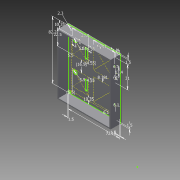
# Autodesk Inventor part: CameraCover
Saved by Autodesk Inventor 2015 (Build 190159000, 159)
## iProperties
Created: 2015-04-23
Part Number: CameraCover
Material: NylonD2W
Document SubType Name: Modeling
Designer: Akovo_000
Density: 1.13 g/cm^3
Appearance: Nylon 6
Mass: 17.9393 g
Surface Area: 219.403 cm^2
Volume: 15.8755 cm^3
Author: Akovo_000
Autodesk Inventor part; units mm, degrees
ref_plane "YZ Plane" through (0, 0, 0) normal (1, 0, 0) x (0, 1, 0)
ref_plane "XZ Plane" through (0, 0, 0) normal (0, 1, 0) x (-1, 0, 0)
ref_plane "XY Plane" through (0, 0, 0) normal (0, 0, 1) x (1, 0, 0)
sketch "Sketch1" plane through (0, 0, 0) normal (0, 1, 0) x (-1, 0, 0)
  line L0 (-58.4836, 42.7915) -> (-27.4836, 42.7915) construction
  line L1 (-27.4836, 42.7915) -> (-27.4836, 11.7915) construction
  line L2 (-27.4836, 11.7915) -> (-58.4836, 11.7915) construction
  line L3 (-58.4836, 11.7915) -> (-58.4836, 20.5915) construction
  line L4 (-58.4836, 42.7915) -> (-27.4836, 11.7915) construction
  line L5 (-27.4836, 42.7915) -> (-58.4836, 11.7915) construction
  line L6 (-58.4836, 3.6103) -> (-27.4836, 3.6103) construction
  line L7 (-27.4836, 3.6103) -> (-27.4836, -27.2085) construction
  line L8 (-27.4836, -27.2085) -> (-58.4836, -27.2085) construction
  line L9 (-58.4836, -27.2085) -> (-58.4836, -18.4991) construction
  line L10 (-58.4836, 3.6103) -> (-27.4836, -27.2085) construction
  line L11 (-20.4336, 38.5415) -> (2.0664, 38.5415) construction
  line L12 (2.0664, 38.5415) -> (2.0664, 16.0415) construction
  line L13 (2.0664, 16.0415) -> (-20.4336, 16.0415) construction
  line L14 (-20.4336, 16.0415) -> (-20.4336, 38.5415) construction
  line L15 (-20.4336, 38.5415) -> (2.0664, 16.0415) construction
  line L16 (2.0664, 38.5415) -> (-20.4336, 16.0415) construction
  line L17 (-20.5481, -0.4585) -> (2.0664, -0.4585) construction
  line L18 (2.0664, -0.4585) -> (2.0664, -22.9585) construction
  line L19 (2.0664, -22.9585) -> (-20.5481, -22.9585) construction
  line L20 (-20.5481, -22.9585) -> (-20.5481, -0.4585) construction
  line L21 (-20.5481, -0.4585) -> (2.0664, -22.9585) construction
  line L22 (2.0664, -0.4585) -> (-20.5481, -22.9585) construction
  line L23 (3.5664, -29.3085) -> (-60.5836, -29.3085) construction
  line L24 (-60.5836, -29.3085) -> (-60.5836, 44.8915) construction
  line L25 (-60.5836, 44.8915) -> (-64.5836, 44.8915) construction
  line L26 (-64.5836, 44.8915) -> (-64.5836, 48.8915)
  line L27 (-64.5836, 48.8915) -> (-60.5836, 48.8915)
  line L28 (-60.5836, 48.8915) -> (-60.5836, 44.8915) construction
  line L29 (-60.5836, -29.3085) -> (-64.5836, -29.3085) construction
  line L30 (-64.5836, -29.3085) -> (-64.5836, -33.3085)
  line L31 (-64.5836, -33.3085) -> (-60.5836, -33.3085)
  line L32 (-60.5836, -33.3085) -> (-60.5836, -29.3085) construction
  line L33 (3.5664, -29.3085) -> (7.5664, -29.3085) construction
  line L34 (7.5664, -29.3085) -> (7.5664, -33.3085)
  line L35 (7.5664, -33.3085) -> (3.5664, -33.3085)
  line L36 (3.5664, -33.3085) -> (3.5664, -29.3085) construction
  line L37 (3.5664, 44.8915) -> (7.5664, 44.8915) construction
  line L38 (7.5664, 44.8915) -> (7.5664, 48.8915)
  line L39 (7.5664, 48.8915) -> (3.5664, 48.8915)
  line L40 (3.5664, 48.8915) -> (3.5664, 44.8915) construction
  circle A0 centre (5.4519, 46.9805) radius 1.15
  circle A1 centre (-62.5836, 46.8915) radius 1.15
  circle A2 centre (-62.5836, -31.3085) radius 1.15
  circle A3 centre (5.5664, -31.3085) radius 1.15
  line L41 (3.5664, 48.8915) -> (-60.5836, 48.8915)
  line L42 (-64.5836, 44.8915) -> (-64.5836, -29.3085)
  line L43 (-60.5836, -33.3085) -> (3.5664, -33.3085)
  line L44 (7.5664, -29.3085) -> (7.5664, 44.8915)
  line L45 (3.5664, 44.8915) -> (-60.5836, 44.8915) construction
  line L46 (3.5664, 44.8915) -> (3.5664, -29.3085) construction
  line L47 (-57.2836, 33.9915) -> (-60.2836, 33.9915)
  line L48 (-60.2836, 33.9915) -> (-60.2836, 20.5915)
  line L49 (-60.2836, 20.5915) -> (-57.2836, 20.5915)
  line L50 (-57.2836, 20.5915) -> (-57.2836, 33.9915)
  line L51 (-57.2836, -5.0991) -> (-60.2836, -5.0991)
  line L52 (-60.2836, -5.0991) -> (-60.2836, -18.4991)
  line L53 (-60.2836, -18.4991) -> (-57.2836, -18.4991)
  line L54 (-57.2836, -18.4991) -> (-57.2836, -5.0991)
  line L55 (-58.4836, 20.5915) -> (-58.4836, 33.9915) construction
  line L56 (-58.4836, 33.9915) -> (-58.4836, 42.7915) construction
  line L57 (-58.4836, -5.0991) -> (-58.4836, 3.6103) construction
  line L58 (-58.4836, -18.4991) -> (-58.4836, -5.0991) construction
  line L59 (-62.5836, 46.8915) -> (-60.5836, 46.8915) construction
  line L60 (-62.5836, 46.8915) -> (-62.5836, 44.8915) construction
  line L61 (-62.5836, 46.8915) -> (-64.5836, 46.8915) construction
  line L62 (-62.5836, 46.8915) -> (-62.5836, 48.8915) construction
  line L63 (-64.5836, -31.3085) -> (-62.5836, -31.3085) construction
  line L64 (-62.5836, -31.3085) -> (-60.5836, -31.3085) construction
  line L65 (-62.5836, -31.3085) -> (-62.5836, -29.3085) construction
  line L66 (-62.5836, -31.3085) -> (-62.5836, -33.3085) construction
  line L67 (5.5664, 46.8915) -> (3.5664, 46.8915) construction
  line L68 (5.5664, 46.8915) -> (7.5664, 46.8915) construction
  line L69 (5.5664, 46.8915) -> (5.5664, 44.8915) construction
  line L70 (5.5664, 44.8915) -> (5.5664, 46.8915) construction
  line L71 (5.5664, 46.8915) -> (5.5664, 48.8915) construction
  line L72 (5.5664, -31.3085) -> (5.5664, -33.3085) construction
  line L73 (5.5664, -31.3085) -> (3.5664, -31.3085) construction
  line L74 (5.5664, -31.3085) -> (5.5664, -29.3085) construction
  line L75 (5.5664, -31.3085) -> (7.5664, -31.3085) construction
  circle A4 centre (-1.9336, 35.5415) radius 2.75
  circle A5 centre (-1.9336, -3.4585) radius 2.75
  line L76 (-1.9336, 35.5415) -> (-1.9336, 38.5415) construction
  line L77 (-1.9336, 35.5415) -> (2.0664, 35.5415) construction
  line L78 (-1.9336, -3.4585) -> (2.0664, -3.4585) construction
  line L79 (-1.9336, -3.4585) -> (-1.9336, -0.4585) construction
  line L80 (-15.9336, 33.9915) -> (-18.9336, 33.9915)
  line L81 (-18.9336, 33.9915) -> (-18.9336, 20.5915)
  line L82 (-18.9336, 20.5915) -> (-15.9336, 20.5915)
  line L83 (-15.9336, 20.5915) -> (-15.9336, 33.9915)
  line L84 (-15.9336, -5.0085) -> (-18.9336, -5.0085)
  line L85 (-18.9336, -5.0085) -> (-18.9336, -18.4085)
  line L86 (-18.9336, -18.4085) -> (-15.9336, -18.4085)
  line L87 (-15.9336, -18.4085) -> (-15.9336, -5.0085)
  line L88 (9.0664, 50.3915) -> (-66.0836, 50.3915)
  line L89 (-66.0836, 50.3915) -> (-66.0836, -34.8085)
  line L90 (-66.0836, -34.8085) -> (9.0664, -34.8085)
  line L91 (9.0664, -34.8085) -> (9.0664, 50.3915)
  point P0 (-89.8981, -75.7195)
  dimension "d0" = 22.5
  dimension "d5" = 31
  dimension "d7" = 22.5
  dimension "d11" = 4
  dimension "d12" = 72.15
  dimension "d13" = 82.2
  dimension "d14" = 2.3
  dimension "d15" = 31
  dimension "d16" = 5.5
  dimension "d17" = 5.5
  dimension "d18" = 10.35
  dimension "d19" = 10.35
  dimension "d20" = 6.1
  dimension "d21" = 6.1
  dimension "d22" = 6.1
  dimension "d23" = 6.1
  dimension "d24" = 3
  dimension "d25" = 13.4
  dimension "d26" = 1.2
  dimension "d27" = 8.1812
  dimension "d28" = 16.5
  dimension "d29" = 5.5
  dimension "d30" = 5.5
  dimension "d31" = 3
  dimension "d32" = 4
  dimension "d33" = 1.5
  dimension "d34" = 4.55
  dimension "d35" = 4.55
  dimension "d36" = 4.55
  dimension "d37" = 1.5
  dimension "d38" = 1.5
  dimension "d39" = 1.5
  dimension "d40" = 1.5
  constraints: 184 end point, 31 parallel, 29 equal length, 20 perpendicular, 15 horizontal, 15 midpoint, 15 point on line, 6 centre point, 4 collinear, 3 equal radius, 3 vertical
  measures "d0" distance of L12.start L12.end
  measures "d5" distance of L1.start L0.start
  measures "d7" distance of L14.end L12.start
  measures "d11" distance of L27.start L27.end
  measures "d12" distance between parallel lines of L30 L34
  measures "d13" distance between parallel lines of L39 L35
  measures "d14" diameter of A0
  measures "d15" distance of L2.end L0.start
  measures "d16" distance from line of L44 L12.end
  measures "d17" distance from line of L44 L18.start
  measures "d18" distance from line of L43 L20.start
  measures "d19" distance between parallel lines of L41 L11
  measures "d20" distance between parallel lines of L41 L0
  measures "d21" distance between parallel lines of L42 L3
  measures "d22" distance between parallel lines of L42 L9
  measures "d23" distance between parallel lines of L43 L8
  measures "d24" distance of L49.end L48.end
  measures "d25" distance of L48.end L47.end
  measures "d26" distance from line of L50 L0.start
  measures "d27" distance between parallel lines of L2 L6
  measures "d28" distance between parallel lines of L13 L17
  measures "d29" diameter of A4
  measures "d30" diameter of A5
  measures "d31" distance of L76.start L76.end
  measures "d32" distance of L76.start L77.end
  measures "d33" distance from line of L81 L14.end
  measures "d34" distance from line of L80 L14.end
  measures "d35" distance between parallel lines of L13 L82
  measures "d36" distance between parallel lines of L84 L17
  measures "d37" distance between parallel lines of L90 L43
  measures "d38" distance between parallel lines of L89 L42
  measures "d39" distance between parallel lines of L88 L41
  measures "d40" distance between parallel lines of L44 L91
extrude "Edges" add sketch "Sketch1" against normal blind 14 contours L91 L90 L89 L88
extrude "Surface" add sketch "Sketch1" along normal blind 1.5 contours L26 L27 L41 L39 L38 L44 L34 L35 L43 L31 L30 L42 | L91 L90 L89 L88
body "Solid1"
